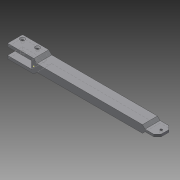
# Autodesk Inventor part: Upper Support beam v2
Saved by Autodesk Inventor 2015 (Build 190159000, 159)
## iProperties
Created: 2019-01-12
Part Number: Upper Support beam v2
Material: Generic
Document SubType Name: Modeling
Designer: Toby
Density: 1 g/cm^3
Appearance: Default
Author: Toby
Autodesk Inventor part; units mm, degrees
ref_plane "YZ Plane" through (0, 0, 0) normal (1, 0, 0) x (0, 1, 0)
ref_plane "XZ Plane" through (0, 0, 0) normal (0, 1, 0) x (-1, 0, 0)
ref_plane "XY Plane" through (0, 0, 0) normal (0, 0, 1) x (1, 0, 0)
sketch "Sketch1" plane through (0, 0, 0) normal (0, 0, 1) x (1, 0, 0)
  line L0 (-83.046, 15.2299) -> (66.954, 15.2299)
  line L1 (66.954, 15.2299) -> (66.954, -4.7701)
  line L2 (66.954, -4.7701) -> (-83.046, -4.7701)
  line L3 (-83.046, -4.7701) -> (-83.046, 15.2299)
  point P0 (0, 0)
  dimension "d0" = 150
  dimension "d1" = 20
  constraints: 8 end point, 2 parallel, 1 horizontal, 1 perpendicular
  measures "d0" distance of L0.start L0.end
  measures "d1" distance of L2.end L0.start
extrude "Extrusion1" add sketch "Sketch1" along normal blind 10
sketch "Sketch2" plane through (-83.046, -4.7701, 0) normal (-1, 0, 0) x (0, 0, 1)
  point P0 (0, 4.7701)
sketch "Sketch3" plane through (-83.046, -4.7701, 0) normal (-1, 0, 0) x (0, 0, 1)
  line L0 (0, 20) -> (-4, 20)
  line L1 (-4, 20) -> (-4, 0)
  line L2 (-4, 0) -> (0, 0)
  line L3 (0, 0) -> (0, 20)
  line L4 (10, 0) -> (14, 0)
  line L5 (14, 0) -> (14, 20)
  line L6 (14, 20) -> (10, 20)
  line L7 (10, 20) -> (10, 0)
  line L8 (0, 0) -> (10, 0) projected
  line L9 (10, 20) -> (10, 0) projected
  point P0 (0, 4.7701)
  dimension "d4" = 4
  dimension "d5" = 4
  constraints: 16 end point, 4 parallel, 2 collinear, 2 horizontal, 2 perpendicular, 2 point on line
  measures "d4" distance of L2.end L1.end
  measures "d5" distance of L6.end L5.end
extrude "Extrusion2" add sketch "Sketch3" against normal blind 5
sketch "Sketch4" plane through (-83.046, -4.7701, 14) normal (-1, 0, 0) x (0, 0, 1)
  line L0 (-18, 20) -> (-14, 20)
  line L1 (-14, 20) -> (-14, 0)
  line L2 (-14, 0) -> (-18, 0)
  line L3 (-18, 0) -> (-18, 20)
  line L4 (0, 20) -> (-4, 20)
  line L5 (-4, 20) -> (-4, 0)
  line L6 (-4, 0) -> (0, 0)
  line L7 (0, 0) -> (0, 20)
  point P0 (-14, 4.7701)
  constraints: 16 end point, 4 parallel, 2 horizontal, 2 perpendicular
extrude "Extrusion3" add sketch "Sketch4" along normal blind 30
sketch "Sketch5" plane through (-78.046, -4.7701, 14) normal (0, 0, 1) x (1, 0, 0)
  line L0 (-35, 0) -> (-35, 20) projected
  line L1 (-5, 20) -> (-35, 20) projected
  line L2 (-5, 0) -> (-5, 20) projected
  point P0 (78.046, 4.7701)
  point P1 (-30, 15)
  point P2 (-10, 15)
  dimension "d10" = 5
  dimension "d11" = 5
  dimension "d12" = 5
  dimension "d13" = 5
  measures "d10" distance from line of L0 point (-30, 15)
  measures "d11" distance from line of L1 point (-30, 15)
  measures "d12" distance from line of L2 point (-10, 15)
  measures "d13" distance from line of L1 point (-10, 15)
hole "Hole1" at (-108.046, 10.2299, 14) at (-88.046, 10.2299, 14) direction (0, 0, -1) diameter 3 depth 30 tip angle 118 countersink diameter 6 countersink angle 90
chamfer "Chamfer1" distance 4 angle 45 2 edges at (-78.046, 5.2299, 10) (-78.046, 5.2299, 0)
sketch "Sketch6" plane through (66.954, -4.7701, 0) normal (0, -1, 0) x (1, 0, 0)
  line L0 (0, -4) -> (-5, -4)
  line L1 (-5, -4) -> (-5, 14)
  line L2 (-5, 14) -> (0, 14)
  line L3 (0, 14) -> (0, -4)
  line L4 (0, 0) -> (-141, 0) projected
  line L5 (-141, 10) -> (0, 10) projected
  line L6 (0, 0) -> (0, 10) projected
  point P0 (-66.954, 0)
  dimension "d24" = 4
  dimension "d25" = 4
  dimension "d26" = 5
  constraints: 8 end point, 2 parallel, 1 collinear, 1 horizontal, 1 perpendicular
  measures "d24" distance between parallel lines of L4 L0
  measures "d25" distance between parallel lines of L5 L2
  measures "d26" distance between parallel lines of L3 L1
extrude "Extrusion4" add sketch "Sketch6" against normal blind 20
sketch "Sketch7" plane through (-113.046, -4.7701, 10) normal (0, -1, 0) x (1, 0, 0)
  line L0 (180, -14) -> (210, -14)
  line L1 (210, -14) -> (210, -10)
  line L2 (210, -10) -> (180, -10)
  line L3 (180, -10) -> (180, -14)
  line L4 (180, 4) -> (210, 4)
  line L5 (210, 4) -> (210, 0)
  line L6 (210, 0) -> (180, 0)
  line L7 (180, 0) -> (180, 4)
  point P0 (113.046, -10)
  dimension "d29" = 30
  dimension "d30" = 30
  dimension "d31" = 4
  dimension "d32" = 4
  constraints: 16 end point, 4 parallel, 2 horizontal, 2 perpendicular
  measures "d29" distance of L2.end L1.end
  measures "d30" distance of L5.end L6.end
  measures "d31" distance of L4.end L5.end
  measures "d32" distance between parallel lines of L0 L2
extrude "Extrusion5" add sketch "Sketch7" against normal blind 20
chamfer "Chamfer2" distance 4 angle 45 2 edges at (61.954, 5.2299, 10) (61.954, 5.2299, 0)
sketch "Sketch8" plane through (96.954, -4.7701, 14) normal (0, 0, 1) x (1, 0, 0)
  line L0 (-30, 20) -> (-30, 0) projected
  line L1 (0, 0) -> (0, 20) projected
  line L2 (-35, 20) -> (0, 20) projected
  line L3 (-35, 0) -> (0, 0) projected
  circle A0 centre (-25, 5) radius 2
  circle A1 centre (-25, 15) radius 2
  circle A2 centre (-5, 5) radius 2
  circle A3 centre (-5, 15) radius 2
  line L4 (-25, 3) -> (-5, 3)
  line L5 (-5, 7) -> (-25, 7)
  line L6 (-25, 13) -> (-5, 13)
  line L7 (-5, 17) -> (-25, 17)
  point P0 (-96.954, 4.7701)
  dimension "d38" = 5
  dimension "d39" = 5
  dimension "d40" = 5
  dimension "d41" = 5
  dimension "d42" = 5
  dimension "d43" = 5
  dimension "d44" = 5
  dimension "d45" = 5
  dimension "d46" = 4
  dimension "d47" = 4
  dimension "d48" = 4
  dimension "d49" = 4
  constraints: 8 end point, 8 point on circle, 4 centre point, 4 coincident, 3 tangent, 1 parallel
  measures "d38" distance from line of L0 point (-25, 5)
  measures "d39" distance from line of L0 point (-25, 15)
  measures "d40" distance from line of L1 point (-5, 5)
  measures "d41" distance from line of L1 point (-5, 15)
  measures "d42" distance from line of L2 point (-25, 15)
  measures "d43" distance from line of L2 point (-5, 15)
  measures "d44" distance from line of L3 point (-25, 5)
  measures "d45" distance from line of L3 point (-5, 5)
  measures "d46" diameter of A0
  measures "d47" diameter of A1
  measures "d48" diameter of A2
  measures "d49" diameter of A3
extrude "Extrusion6" cut sketch "Sketch8" against normal blind 20 contours A0 | A0 L5 A2 L4 | A2 | A1 | A1 L7 A3 L6 | A3
sketch "Sketch9" plane through (-113.046, -4.7701, 10) normal (0, -1, 0) x (1, 0, 0)
  line L0 (30, -10) -> (31.8516, -10)
  line L1 (31.8516, -10) -> (31.8516, 0)
  line L2 (31.8516, 0) -> (30, 0)
  line L3 (30, 0) -> (30, -10)
  line L4 (30, 0) -> (0, 0) projected
  point P0 (113.046, -10)
  dimension "d52" = 1.8516
  constraints: 8 end point, 2 parallel, 1 collinear, 1 horizontal, 1 perpendicular
  measures "d52" distance between parallel lines of L3 L1
extrude "Extrusion7" cut sketch "Sketch9" against normal blind 20
sketch "Sketch10" plane through (-113.046, 15.2299, 14) normal (0, 1, 0) x (1, 0, 0)
  line L0 (171, 4) -> (210, 4)
  line L1 (210, 4) -> (210, 0)
  line L2 (210, 0) -> (171, 0)
  line L3 (171, 0) -> (171, 4)
  line L4 (210, 18) -> (171, 18)
  line L5 (171, 18) -> (171, 14)
  line L6 (171, 14) -> (210, 14)
  line L7 (210, 14) -> (210, 18)
  line L8 (180, 14) -> (210, 14) projected
  point P0 (113.046, 14)
  constraints: 16 end point, 4 parallel, 2 horizontal, 2 perpendicular, 1 collinear, 1 point on line
extrude "Extrusion8" cut sketch "Sketch10" against normal blind 20
sketch "Sketch11" plane through (66.954, 15.2299, 10) normal (0, 1, 0) x (1, 0, 0)
  line L0 (0, 0) -> (0, 10) projected
  line L1 (0, 3.5) -> (20, 3.5)
  line L2 (20, 3.5) -> (20, 6.5)
  line L3 (20, 6.5) -> (0, 6.5)
  line L4 (0, 6.5) -> (0, 3.5)
  line L5 (0, 0) -> (-141, 0) projected
  point P0 (-66.954, 10)
  dimension "d57" = 3
  dimension "d58" = 3.5
  dimension "d59" = 20
  constraints: 8 end point, 2 parallel, 1 horizontal, 1 perpendicular, 1 point on line
  measures "d57" distance between parallel lines of L3 L1
  measures "d58" distance between parallel lines of L5 L1
  measures "d59" distance between parallel lines of L0 L2
extrude "Extrusion9" add sketch "Sketch11" against normal blind 20
sketch "Sketch12" plane through (66.954, 15.2299, 6.5) normal (0, 0, 1) x (1, 0, 0)
  line L0 (20, -20) -> (0, -20) projected
  line L1 (20, 0) -> (20, -20) projected
  point P0 (-66.954, -15.2299)
  point P1 (15, -10)
  dimension "d62" = 10
  dimension "d63" = 5
  measures "d62" distance from line of L0 point (15, -10)
  measures "d63" distance from line of L1 point (15, -10)
hole "Hole2" at (81.954, 5.2299, 6.5) direction (0, 0, -1) diameter 3 depth 8 tip angle 118
chamfer "Chamfer3" distance 5 angle 45 2 edges at (86.954, -4.7701, 5) (86.954, 15.2299, 5)
chamfer "Chamfer4" distance 3.5 angle 45 2 edges at (66.954, 5.2299, 6.5) (66.954, 5.2299, 3.5)
body "Solid1"
